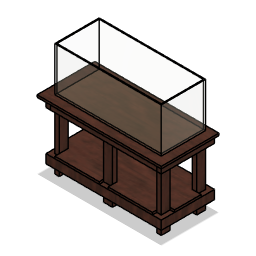
Aquario v1 (Autodesk Fusion 360 design; units mm, degrees)
Autodesk Fusion 360 part; units mm, degrees
note: some values were not read from the file. Set by a fixed rule: which sketch regions a step uses.
sketch "Sketch1" plane through (0, 0, 0) normal (0, 1, 0) x (1, 0, 0)
  line L0 (0, 0) -> (50, 0)
  line L1 (50, 0) -> (50, -100)
  line L2 (50, -100) -> (0, -100)
  line L3 (0, -100) -> (0, 0)
  line L4 (1150, -100) -> (1150, 0)
  line L5 (1150, 0) -> (1200, 0)
  line L6 (1200, 0) -> (1200, -100)
  line L7 (1200, -100) -> (1150, -100)
  line L8 (0, -500) -> (0, -400)
  line L9 (0, -400) -> (50, -400)
  line L10 (50, -400) -> (50, -500)
  line L11 (50, -500) -> (0, -500)
  line L12 (1150, -500) -> (1150, -400)
  line L13 (1150, -400) -> (1200, -400)
  line L14 (1200, -400) -> (1200, -500)
  line L15 (1200, -500) -> (1150, -500)
  line L16 (550, 0) -> (650, 0)
  line L17 (650, 0) -> (650, -50)
  line L18 (650, -50) -> (550, -50)
  line L19 (550, -50) -> (550, 0)
  line L20 (550, -450) -> (650, -450)
  line L21 (650, -450) -> (650, -500)
  line L22 (650, -500) -> (550, -500)
  line L23 (550, -500) -> (550, -450)
  line L24 (600, 92.4103) -> (600, -713.1129) construction
  dimension "d1" = 100
  dimension "d2" = 50
  dimension "d5" = 1150
  dimension "d6" = -400
  dimension "d7" = 1200
  dimension "d8" = 500
  constraint horizontal L0
  constraint vertical L1
  constraint horizontal L2
  constraint vertical L3
  constraint coincident L0.start L3.end
  constraint horizontal L16
  constraint vertical L17
  constraint horizontal L18
  constraint vertical L19
  constraint horizontal L20
  constraint vertical L21
  constraint horizontal L22
  constraint vertical L23
  constraint perpendicular L18 L24
  constraint symmetric L3 L6 L24
  constraint collinear L19 L23
  constraint collinear L17 L21
  constraint equal L6 L18
  constraint equal L5 L17
  constraint collinear L5 L16
  constraint collinear L15 L22
  constraint equal L17 L21
  measures "d1" distance of L0.start L2.end
  measures "d2" distance of L0.start L0.end
  measures "d7" distance of L3 L6
  measures "d8" distance of L0 L11
extrude "Extrude1" add sketch "Sketch1" along normal blind 750 makes body 1 at (50, 250, 33.3333) makes body 2 at (0, 250, 466.6667) makes body 3 at (1150, 250, 66.6667) makes body 4 at (1150, 250, 466.6667) makes body 5 at (583.3333, 250, 0) makes body 6 at (616.6667, 250, 500)
ref_plane "WorkPlane1" through (25, 750, 450) normal (0, 1, 0) x (0, 0, 1)
sketch "Tampo" plane through (25, 750, 450) normal (0, 1, 0) x (1, 0, 0)
  line L0 (-125, 500) -> (1275, 500)
  line L1 (1275, 500) -> (1275, -150)
  line L2 (1275, -150) -> (-125, -150)
  line L3 (-125, -150) -> (-125, 500)
  point P0 (-25, -50)
  point P1 (-25, 450)
  point P2 (1175, 450)
  point P3 (1175, -50)
  dimension "d12" = 100
  dimension "d13" = 50
  dimension "d14" = 100
  dimension "d15" = 100
  constraint horizontal L0
  constraint vertical L1
  constraint horizontal L2
  constraint vertical L3
  measures "d12" distance of P0 L2
  measures "d13" distance of P1 L0
  measures "d14" distance of P1 L3
  measures "d15" distance of P2 L1
extrude "Extrude2" add sketch "Tampo" along normal blind 25 separate body makes body 7
sketch "Sketch7" plane through (1200, 0, 0) normal (1, 0, 0) x (0, 0, -1)
  line L0 (-500, 0) -> (-400, 0)
  line L1 (-400, 0) -> (-400, 750)
  line L2 (-400, 750) -> (-500, 750)
  line L3 (-500, 750) -> (-500, 0)
  line L4 (-500, 750) -> (-550, 750)
  line L5 (-550, 750) -> (-550, 650)
  line L6 (-550, 650) -> (-500, 650)
  line L7 (-500, 650) -> (-500, 750)
  line L8 (-600, 775) -> (50, 775)
  line L9 (-100, 0) -> (0, 0)
  line L10 (0, 0) -> (0, 750)
  line L11 (0, 750) -> (-100, 750)
  line L12 (-100, 750) -> (-100, 0)
  line L13 (0, 650) -> (50, 650)
  line L14 (50, 750) -> (-600, 750)
  line L15 (50, 650) -> (50, 750)
  dimension "d18" = 50
  dimension "d19" = 100
  dimension "d22" = 50
  dimension "d23" = 100
  constraint horizontal L4
  constraint vertical L5
  constraint horizontal L6
  constraint vertical L7
  constraint coincident L2.end L3.start
  constraint coincident L10 L13.start
  constraint perpendicular L10 L13
  constraint coincident L14 L15.end
  constraint perpendicular L14 L15
  measures "d18" distance of L5.end L6.end
  measures "d19" distance of L4.end L5.end
  measures "d22" distance of L13.start L13.end
  measures "d23" distance of L13.end L14.start
extrude "Extrude3" add sketch "Sketch7" against normal up to surface (1200 mm away) separate body contours L3 L4 L5 L6 L7 L14 | L10 L13 L14 L15 makes body 8 at (800, 716.6667, 550) makes body 9 at (800, 683.3333, 0)
sketch "Sketch8" plane through (0, 0, 550) normal (0, 0, 1) x (1, 0, 0)
  line L0 (0, 750) -> (0, 650)
  line L1 (0, 650) -> (1200, 650)
  line L2 (1200, 650) -> (1200, 750)
  line L3 (1200, 750) -> (0, 750)
  line L4 (1200, 650) -> (1250, 650)
  line L5 (1250, 650) -> (1250, 750)
  line L6 (1250, 750) -> (1200, 750)
  line L7 (1200, 750) -> (1200, 650)
  line L8 (0, 650) -> (-50, 650)
  line L9 (-50, 650) -> (-50, 750)
  line L10 (-50, 750) -> (0, 750)
  line L11 (0, 750) -> (0, 650)
  line L12 (1300, 750) -> (-100, 750)
  dimension "d24" = 50
  dimension "d25" = 50
  constraint horizontal L4
  constraint vertical L5
  constraint horizontal L6
  constraint vertical L7
  constraint coincident L1.end L2.start
  constraint horizontal L8
  constraint vertical L9
  constraint horizontal L10
  constraint vertical L11
  constraint coincident L0.end L1.start
  constraint coincident L10 L12.end
  constraint coincident L6 L12.start
  measures "d24" distance of L1.end L4.end
  measures "d25" distance of L0.end L8.end
extrude "Extrude4" add sketch "Sketch8" against normal up to surface (600 mm away) separate body contours L0 L8 L9 L10 L11 L12 | L2 L4 L5 L6 L7 L12 makes body 10 at (0, 716.6667, 350) makes body 11 at (1250, 683.3333, 350)
extrude "Extrude5" add 4 faces at (1216.6667, 650, 350) (800, 650, 533.3333) (800, 650, -16.6667) (-16.6667, 650, 350) along direction (0, 1, 0) blind 100 from surface at 100 separate body start surface through (0, 0, 0) normal (0, -1, 0) on bodies 8 9 10 11 makes body 12
sketch "Vidro" plane through (0, 775, 0) normal (0, 1, 0) x (-1, 0, 0)
  line L0 (100, 600) -> (-1300, 600)
  line L1 (-1300, 600) -> (-1300, -50)
  line L2 (-1300, -50) -> (100, -50)
  line L3 (100, -50) -> (100, 600)
  line L4 (0, 0) -> (-1200, 0)
  line L5 (-1200, 0) -> (-1200, 500)
  line L6 (-1200, 500) -> (0, 500)
  line L7 (0, 500) -> (0, 0)
  line L8 (-1188, 488) -> (-12, 488)
  line L9 (-12, 488) -> (-12, 12)
  line L10 (-12, 12) -> (-1188, 12)
  line L11 (-1188, 12) -> (-1188, 488)
  dimension "d31" = 50
  dimension "d32" = 100
  dimension "d33" = 100
  dimension "d34" = 100
  dimension "d35" = 12
  constraint horizontal L4
  constraint vertical L5
  constraint horizontal L6
  constraint vertical L7
  measures "d31" distance of L2 L4
  measures "d32" distance of L0 L6
  measures "d33" distance of L3 L7
  measures "d34" distance of L1 L5
extrude "Extrude6" add sketch "Vidro" along normal blind 12 separate body contours L8 L9 L10 L11 makes body 13
extrude "Extrude7" add sketch "Vidro" along normal blind 500 contours L4 L5 L6 L7 bodies 13
sketch "Sketch10" plane through (0, 200, 0) normal (0, 1, 0) x (-1, 0, 0)
  line L0 (0, 0) -> (-1200, 0)
  line L1 (-1200, 0) -> (-1200, 500)
  line L2 (-1200, 500) -> (0, 500)
  line L3 (0, 500) -> (0, 0)
  line L4 (-1250, -50) -> (50, -50)
  line L5 (50, -50) -> (50, 550)
  line L6 (50, 550) -> (-1250, 550)
  line L7 (-1250, 550) -> (-1250, -50)
  line L8 (0, 100) -> (-50, 100)
  line L9 (-50, 100) -> (-50, 0)
  line L10 (-50, 0) -> (0, 0)
  line L11 (0, 0) -> (0, 100)
  line L12 (-50, 500) -> (-50, 400)
  line L13 (-50, 400) -> (0, 400)
  line L14 (0, 400) -> (0, 500)
  line L15 (0, 500) -> (-50, 500)
  line L16 (-550, 50) -> (-650, 50)
  line L17 (-650, 50) -> (-650, 0)
  line L18 (-650, 0) -> (-550, 0)
  line L19 (-550, 0) -> (-550, 50)
  line L20 (-550, 500) -> (-650, 500)
  line L21 (-650, 500) -> (-650, 450)
  line L22 (-650, 450) -> (-550, 450)
  line L23 (-550, 450) -> (-550, 500)
  line L24 (-1200, 100) -> (-1200, 0)
  line L25 (-1200, 0) -> (-1150, 0)
  line L26 (-1150, 0) -> (-1150, 100)
  line L27 (-1150, 100) -> (-1200, 100)
  line L28 (-1200, 500) -> (-1200, 400)
  line L29 (-1200, 400) -> (-1150, 400)
  line L30 (-1150, 400) -> (-1150, 500)
  line L31 (-1150, 500) -> (-1200, 500)
  line L32 (0, 100) -> (50, 100)
  line L33 (-50, 0) -> (-50, -50)
  line L34 (0, 400) -> (50, 400)
  line L35 (-50, 500) -> (-50, 550)
  line L36 (-1150, 0) -> (-1150, -50)
  line L37 (-1200, 100) -> (-1250, 100)
  line L38 (-1200, 400) -> (-1250, 400)
  line L39 (-1150, 500) -> (-1150, 550)
  line L40 (-550, 0) -> (-550, -50)
  line L41 (-650, 0) -> (-650, -50)
  line L42 (-550, 500) -> (-550, 550)
  line L43 (-650, 500) -> (-650, 550)
  constraint coincident L8.start L11.end
  constraint coincident L5 L32.end
  constraint perpendicular L5 L32
  constraint coincident L9.end L10.start
  constraint coincident L4 L33.end
  constraint perpendicular L4 L33
  constraint coincident L13.end L14.start
  constraint coincident L5 L34.end
  constraint perpendicular L5 L34
  constraint coincident L12.start L15.end
  constraint coincident L6 L35.end
  constraint perpendicular L6 L35
  constraint coincident L25.end L26.start
  constraint coincident L4 L36.end
  constraint perpendicular L4 L36
  constraint coincident L24.start L27.end
  constraint coincident L7 L37.end
  constraint perpendicular L7 L37
  constraint coincident L28.end L29.start
  constraint perpendicular L28 L38
  constraint coincident L30.end L31.start
  constraint coincident L6 L39.end
  constraint perpendicular L6 L39
  constraint coincident L7 L38.end
  constraint coincident L18.end L19.start
  constraint coincident L4 L40.end
  constraint perpendicular L4 L40
  constraint coincident L17.end L18.start
  constraint coincident L4 L41.end
  constraint perpendicular L4 L41
  constraint coincident L20.start L23.end
  constraint coincident L6 L42.end
  constraint perpendicular L6 L42
  constraint coincident L20.end L21.start
  constraint coincident L6 L43.end
  constraint perpendicular L6 L43
extrude "Extrude8" add sketch "Sketch10" along normal blind 25 separate body contours L0 L4 L33 L40 | L0 L1 L2 L3 L8 L9 L12 L13 L16 L17 L19 L21 L22 L23 L26 L27 L29 L30 | L3 L5 L32 L34 | L0 L4 L36 L41 | L2 L6 L35 L42 | L1 L7 L37 L38 | L2 L6 L39 L43 makes body 14
named bodies: "Saiote", "Tampo Tampo", "Aquario", "Tambo Base"
